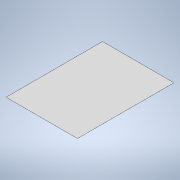
# Autodesk Inventor part: Paper
Saved by Autodesk Inventor 2021 (Build 250183000, 183)
## iProperties
Created: 2022-03-13
Part Number: Paper
Material: Generic
Document SubType Name: Modeling
Designer: stefi
Density: 1 g/cm^3
Appearance: Default
Author: stefi
Autodesk Inventor part; units mm, degrees
ref_plane "YZ Plane" through (0, 0, 0) normal (1, 0, 0) x (0, 1, 0)
ref_plane "XZ Plane" through (0, 0, 0) normal (0, 1, 0) x (-1, 0, 0)
ref_plane "XY Plane" through (0, 0, 0) normal (0, 0, 1) x (1, 0, 0)
sketch "Sketch1" plane through (0, 0, 0) normal (0, 1, 0) x (-1, 0, 0)
  line L0 (254, -342.9) -> (-254, -342.9)
  line L1 (-254, -342.9) -> (-254, 342.9)
  line L2 (-254, 342.9) -> (254, 342.9)
  line L3 (254, 342.9) -> (254, -342.9)
  line L4 (254, -342.9) -> (-254, 342.9) construction
  line L5 (-254, -342.9) -> (254, 342.9) construction
  point P0 (0, 0)
  dimension "d0" = 508
  dimension "d1" = 685.8
  constraints: 12 end point, 2 midpoint, 2 parallel, 1 horizontal, 1 perpendicular
  measures "d0" distance of L1.end L2.end
  measures "d1" distance of L0.end L1.end
extrude "Extrusion1" add sketch "Sketch1" along normal blind 0.127
body "Solid1"
